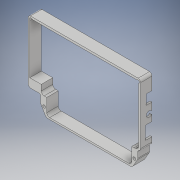
# Autodesk Inventor part: Casing
Saved by Autodesk Inventor 2019.4 (Build 234330000, 330)
## iProperties
Created: 2020-08-29
Part Number: Casing
Material: Generic
Document SubType Name: Modeling
Designer: craig
Density: 1 g/cm^3
Appearance: Default
Author: craig
## iProperties of the stored document _3DPrint.ipt
Created: 2020-09-16
Part Number: _3DPrint
Material: Generic
Document SubType Name: Modeling
Designer: craig
Density: 1 g/cm^3
Appearance: Default
Author: craig
Autodesk Inventor part; units mm, degrees
ref_plane "YZ Plane" through (0, 0, 0) normal (1, 0, 0) x (0, 1, 0)
ref_plane "XZ Plane" through (0, 0, 0) normal (0, 1, 0) x (-1, 0, 0)
ref_plane "XY Plane" through (0, 0, 0) normal (0, 0, 1) x (1, 0, 0)
sketch "Sketch7" plane through (0, 0, 0) normal (0, 0, 1) x (1, 0, 0)
  line L0 (92.45, -34.85) -> (92.2893, -34.85) projected
  line L1 (92.2893, -34.85) -> (92.2893, -46.3269) projected
  line L2 (92.2893, -46.3269) -> (83.2555, -46.3269) projected
  line L3 (83.2555, -46.3269) -> (83.2555, -34.85) projected
  line L4 (83.2555, -34.85) -> (-64.8533, -34.85) projected
  line L5 (-64.8533, -34.85) -> (-64.8533, -45.8213) projected
  line L6 (-64.8533, -45.8213) -> (-73.8416, -45.8213) projected
  line L7 (-73.8416, -45.8213) -> (-73.8416, -34.85) projected
  line L8 (-73.8416, -34.85) -> (-74.45, -34.85) projected
  line L9 (-74.45, -34.85) -> (-74.45, -19.925) projected
  line L10 (-74.45, -19.925) -> (-94.45, -19.925) projected
  line L11 (-94.45, -19.925) -> (-94.45, 66.85) projected
  line L12 (-94.45, 66.85) -> (-93.95, 66.85) projected
  arc A0 (-90.0713, 69.6192) -> (-93.95, 66.85) centre (-92.45, 68.85) ccw projected
  arc A1 (-90.0713, 69.6192) -> (-86.2653, 66.85) centre (-86.2653, 70.85) ccw projected
  line L13 (-86.2653, 66.85) -> (-73.2725, 66.85) projected
  line L14 (-73.2725, 66.85) -> (-73.2725, 70.4275) projected
  line L15 (-73.2725, 70.4275) -> (92.6104, 70.4275) projected
  arc A2 (95.0772, 66.1658) -> (92.6104, 70.4275) centre (94.2193, 68.514) ccw projected
  arc A3 (95.0772, 66.1658) -> (92.45, 62.4088) centre (96.45, 62.4088) ccw projected
  line L16 (92.45, 62.4088) -> (92.45, -34.85) projected
  arc A4 (98.45, 68.85) -> (94.45, 72.85) centre (94.45, 68.85) ccw projected
  line L17 (94.45, 72.85) -> (-93.45, 72.85) projected
  arc A5 (-93.45, 72.85) -> (-97.45, 68.85) centre (-93.45, 68.85) ccw projected
  line L18 (-97.45, 68.85) -> (-97.45, -35.0582) projected
  line L19 (-97.45, -35.0582) -> (-78, -35.0582) projected
  line L20 (96, -35.0582) -> (98.45, -35.0582) projected
  line L21 (98.45, -35.0582) -> (98.45, 68.85) projected
  arc A6 (-76, -37.0582) -> (-78, -35.0582) centre (-78, -37.0582) ccw projected
  line L22 (-76, -37.0582) -> (-76, -48.5295) projected
  line L23 (-66, -65.85) -> (84, -65.85) projected
  line L24 (94, -48.5295) -> (94, -37.0582) projected
  arc A7 (96, -35.0582) -> (94, -37.0582) centre (96, -37.0582) ccw projected
  circle A8 centre (-69.3475, -50.8213) radius 2.5 projected
  circle A9 centre (87.7724, -50.8213) radius 2.5 projected
  line L25 (94, -48.5295) -> (84, -65.85) projected
  line L26 (-66, -65.85) -> (-76, -48.5295) projected
  point P0 (0, 0)
  point P1 (-74.5366, -65.85)
  point P2 (92.6375, -65.85)
extrude "Extrusion6" add sketch "Sketch7" along normal blind 20 contours L21 L20 A7 L24 L25 L23 L26 L22 A6 L19 L18 A5 L17 A4 | A8 | A9
sketch "Sketch8" plane through (0, 0, 20) normal (0, 0, 1) x (1, 0, 0)
  line L0 (-64.8533, -34.85) -> (83.2555, -34.85)
  line L1 (83.2555, -34.85) -> (83.2555, -62.85)
  line L2 (83.2555, -62.85) -> (-64.8533, -62.85)
  line L3 (-64.8533, -62.85) -> (-64.8533, -34.85)
  line L4 (-66, -65.85) -> (84, -65.85) projected
  point P0 (0, 0)
  point P1 (-76, -65.85)
  point P2 (94, -65.85)
  dimension "d19" = 3
  constraints: 8 end point, 2 coincident, 2 parallel, 1 horizontal, 1 perpendicular
  measures "d19" distance between parallel lines of L4 L2
sketch "Sketch9" plane through (0, 0, 20) normal (0, 0, 1) x (1, 0, 0)
  line L0 (-73.2725, 70.4275) -> (91.6133, 70.4275)
  line L1 (91.6133, 70.4275) -> (91.6133, 67.0798)
  line L2 (91.6133, 67.0798) -> (-73.2725, 67.0798)
  line L3 (-73.2725, 67.0798) -> (-73.2725, 70.4275)
  point P0 (0, 0)
  constraints: 8 end point, 2 parallel, 1 coincident, 1 horizontal, 1 perpendicular
extrude "Extrusion8" add sketch "Sketch9" against normal up to surface (20 mm away)
fillet "Fillet3" radius 2 1 edges at (91.6133, 70.4275, 10)
sketch "Sketch10" plane through (0, 0, 20) normal (0, 0, 1) x (1, 0, 0)
  line L0 (-73.8416, -34.85) -> (-64.8533, -34.85)
  line L1 (-64.8533, -34.85) -> (-64.8533, -45.8213)
  line L2 (-64.8533, -45.8213) -> (-73.8416, -45.8213)
  line L3 (-73.8416, -45.8213) -> (-73.8416, -34.85)
  line L4 (83.2555, -34.85) -> (92.2893, -34.85)
  line L5 (92.2893, -34.85) -> (92.2893, -46.3269)
  line L6 (92.2893, -46.3269) -> (83.2555, -46.3269)
  line L7 (83.2555, -46.3269) -> (83.2555, -34.85)
  point P0 (0, 0)
  constraints: 16 end point, 4 coincident, 4 parallel, 2 horizontal, 2 perpendicular
extrude "Extrusion9" add sketch "Sketch10" against normal up to surface (20 mm away)
extrude "Extrusion10" cut sketch "Sketch8" against normal up to surface (20 mm away)
fillet "Fillet4" radius 5 4 edges at (-74.45, -34.85, 10) (-64.8533, -62.85, 10) (83.2555, -62.85, 10) (92.45, -34.85, 10)
sketch "Sketch11" plane through (0, 0, 20) normal (0, 0, 1) x (1, 0, 0)
  circle A0 centre (-69.3475, -50.8213) radius 2.5 projected
  circle A1 centre (87.7724, -50.8213) radius 2.5 projected
  point P0 (0, 0)
extrude "Extrusion11" cut sketch "Sketch11" against normal up to surface (20 mm away)
fillet "Fillet5" radius 5 6 edges at (98.45, -35.0582, 10) (94, -48.5295, 10) (84, -65.85, 10) (-66, -65.85, 10) (-76, -48.5295, 10) (-97.45, -35.0582, 10)
sketch "Sketch15" plane through (0, 0, 20) normal (0, 0, 1) x (1, 0, 0)
  arc A0 (95.0772, 66.1658) -> (92.6104, 70.4275) centre (94.2193, 68.514) ccw projected
  arc A1 (92.6104, 70.4275) -> (95.0772, 66.1658) centre (94.2193, 68.514) ccw
  point P0 (0, 0)
  constraints: 2 point on circle, 1 centre point, 1 concentric
extrude "Extrusion14" cut sketch "Sketch15" against normal blind 2
sketch "Sketch16" plane through (0, 0, 20) normal (0, 0, 1) x (1, 0, 0)
  arc A0 (98.45, 68.85) -> (94.45, 73.85) centre (93.7112, 69.159) ccw projected
  line L0 (-93.45, 73.85) -> (94.45, 73.85) projected
  line L1 (94.45, 72.85) -> (-93.45, 72.85) projected
  arc A1 (98.45, 68.85) -> (94.45, 72.85) centre (94.45, 68.85) ccw projected
  arc A2 (-93.45, 73.85) -> (-97.45, 68.85) centre (-92.7112, 69.159) ccw projected
  arc A3 (-93.45, 72.85) -> (-97.45, 68.85) centre (-93.45, 68.85) ccw projected
  point P0 (0, 0)
extrude "Extrusion15" add sketch "Sketch16" against normal up to surface (20 mm away)
sketch "Sketch17" plane through (0, 0, 20) normal (0, 0, 1) x (1, 0, 0)
  line L0 (-92.1356, 70.139) -> (95.2506, 70.139)
  line L1 (95.2506, 70.139) -> (95.2506, -33.7438)
  line L2 (95.2506, -33.7438) -> (43.7025, -33.7438)
  line L3 (43.7025, -33.7438) -> (-92.1356, 70.139)
  point P0 (0, 0)
  constraints: 8 end point, 2 perpendicular, 1 horizontal
extrude "Extrusion16" cut sketch "Sketch17" against normal up to surface (20 mm away)
fillet "Fillet6" radius 4 1 edges at (95.2506, -33.7438, 10)
sketch "Sketch18" plane through (98.45, -30.5392, 20) normal (1, 0, 0) x (0, 0, -1)
  line L0 (20, 31.0685) -> (8, 31.0685)
  line L1 (8, 31.0685) -> (8, 8.0685)
  line L2 (8, 8.0685) -> (20, 8.0685)
  line L3 (20, 8.0685) -> (20, 31.0685)
  line L4 (20, 0) -> (20, 99.3892) projected
  point P0 (20, 30.5392)
  dimension "d46" = 23
  dimension "d47" = 12
  constraints: 8 end point, 2 parallel, 1 horizontal, 1 perpendicular, 1 point on line
  measures "d46" distance of L0.end L1.end
  measures "d47" distance of L0.start L0.end
extrude "Extrusion17" cut sketch "Sketch18" against normal blind 10
sketch "Sketch19" plane through (98.45, -30.5392, 20) normal (1, 0, 0) x (0, 0, -1)
  circle A0 centre (15.1, 44.8724) radius 5
  line L0 (20, 31.0685) -> (20, 99.3892) projected
  point P0 (20, 30.5392)
  dimension "d50" = 10
  dimension "d59" = 4.9
  constraints: 1 centre point
  measures "d50" diameter of A0
  measures "d59" distance from line of L0 A0.centre
extrude "Extrusion18" cut sketch "Sketch19" against normal blind 10
sketch "Sketch20" plane through (98.45, -30.5392, 20) normal (1, 0, 0) x (0, 0, -1)
  line L0 (20, 77.5481) -> (9.7, 77.5481)
  line L1 (9.7, 77.5481) -> (9.7, 60.3481)
  line L2 (9.7, 60.3481) -> (20, 60.3481)
  line L3 (20, 60.3481) -> (20, 77.5481)
  line L4 (20, 0) -> (20, 99.3892) projected
  point P0 (20, 30.5392)
  point P1 (20, 44.8724)
  dimension "d53" = 10.3
  dimension "d54" = 17.2
  constraints: 8 end point, 2 parallel, 1 horizontal, 1 perpendicular, 1 point on line
  measures "d53" distance of L0.start L0.end
  measures "d54" distance of L0.end L1.end
extrude "Extrusion19" cut sketch "Sketch20" against normal blind 10
fillet "Fillet7" radius 2 2 edges at (96.8503, 0.5293, 12) (96.8503, -22.4707, 12)
fillet "Fillet8" radius 1 2 edges at (96.8503, 29.8088, 10.3) (96.8503, 47.0088, 10.3)
fillet "Fillet9" radius 0.5 2 edges at (96.8503, 13.3382, 0) (96.8503, 15.3282, 0)
body "Solid4"
